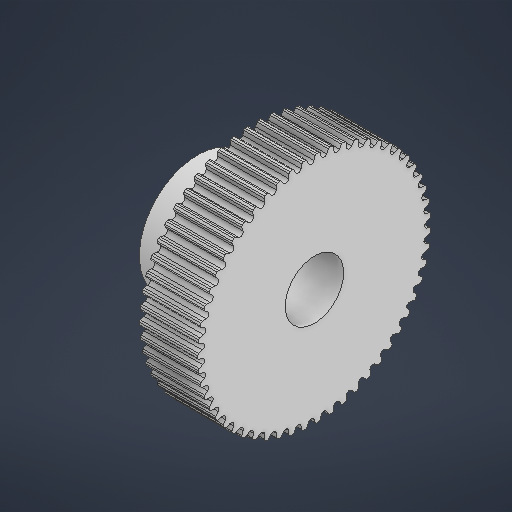
# Autodesk Inventor part: P_Zahnrad
Saved by Autodesk Inventor 2026 (Build 300175000, 175)
## iProperties
Created: 2025-04-26
Part Number: P_Zahnrad
Material: Generisch
Document SubType Name: Modeling
Designer: FAL
Density: 1 g/cm^3
Appearance: Vorgabe
Author: FAL
Autodesk Inventor part; units mm, degrees
ref_plane "YZ Plane" through (0, 0, 0) normal (1, 0, 0) x (0, 1, 0)
ref_plane "XZ Plane" through (0, 0, 0) normal (0, 1, 0) x (-1, 0, 0)
ref_plane "XY Plane" through (0, 0, 0) normal (0, 0, 1) x (1, 0, 0)
sketch "Skizze1" plane through (0, 0, 0) normal (0, 0, 1) x (1, 0, 0)
  line L0 (0, 2) -> (0, 4)
  line L1 (0, 4) -> (4, 4)
  line L2 (4, 4) -> (4, 8)
  line L3 (4, 8) -> (8, 8)
  line L4 (8, 8) -> (8, 2)
  line L5 (7.4579, 0) -> (0, 0)
  line L6 (0, 2) -> (8, 2)
  line L7 (0, -1.6) -> (0, 9.6) projected
  point P0 (6, 8)
  dimension "d0" = 4
  dimension "d1" = 8
  dimension "d2" = 16
  dimension "d3" = 4
  dimension "d4" = 4
  constraints: 14 end point, 6 perpendicular, 1 collinear, 1 midpoint, 1 vertical
  measures "d0" diameter of L6 L5
  measures "d1" diameter of L1 L5
  measures "d2" diameter of point (6, 8) L5
  measures "d3" distance between parallel lines of L0 L2
  measures "d4" distance between parallel lines of L4 L2
revolve "Umdrehung1" add sketch "Skizze1" angle 360 about axis through (7.4579, 0, 0) along (-1, 0, 0)
sketch "Skizze2" plane through (0, 0, 0) normal (1, 0, 0) x (0, 1, 0)
  arc A0 (7.679, 0.187) -> (7.55, 0) centre (7.75, 0) ccw
  line L0 (7.679, 0.187) -> (8.2403, 0.4)
  line L1 (7.55, 0) -> (8.25, 0)
  arc A1 (8.25, 0) -> (8.2403, 0.4) centre (0, 0) ccw
  arc A2 (7.55, 0) -> (7.679, -0.187) centre (7.75, 0) ccw
  line L2 (7.679, -0.187) -> (8.2403, -0.4)
  arc A3 (8.2403, -0.4) -> (8.25, 0) centre (0, 0) ccw
  circle A4 centre (0, 0) radius 7.75 construction
  circle A5 centre (0, 0) radius 2 projected
  dimension "d10" = 15.5
  dimension "d11" = 0.2
  dimension "d12" = 0.5
  dimension "d13" = 0.4
  constraints: 8 point on circle, 6 end point, 4 centre point, 2 symmetric about line, 1 coincident, 1 horizontal, 1 horizontal alignment, 1 point on line, 1 tangent, 5 other
  measures "d11" radius of A0
  measures "d12" distance of A0.centre L1.end
  measures "d13" vertical distance of L1.end L0.end
extrude "Extrusion1" cut sketch "Skizze2" along normal blind 10 contours L0 A1 L1 A0 | L1 A3 L2 A2
fillet "Rundung1" radius 0.1 2 edges at (6, 7.9941, -0.3066) (6, 7.9941, 0.3066)
pattern_circular "Runde Anordnung1" count 55 over 360 about axis through (-10, 0, 0) along (1, 0, 0) of "Rundung1", "Extrusion1"
